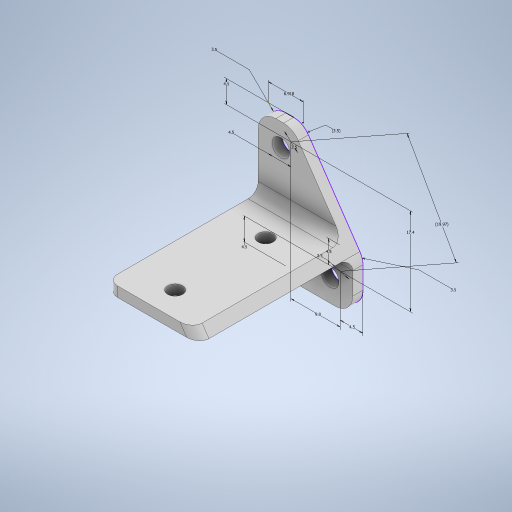
# Autodesk Inventor part: BLTouch Mount
Saved by Autodesk Inventor 2023 (Build 270158000, 158)
## iProperties
Created: 2024-01-21
Part Number: BLTouch Mount
Material: Generic
Document SubType Name: Modeling
Designer: Lyall
Density: 1 g/cm^3
Appearance: Default
Author: Lyall
Autodesk Inventor part; units mm, degrees
note: some values were not read from the file. Chosen so that the rebuilt part matches the saved one: edges of "Fillet2".
ref_plane "YZ Plane" through (0, 0, 0) normal (1, 0, 0) x (0, 1, 0)
ref_plane "XZ Plane" through (0, 0, 0) normal (0, 1, 0) x (-1, 0, 0)
ref_plane "XY Plane" through (0, 0, 0) normal (0, 0, 1) x (1, 0, 0)
sketch "Sketch1" plane through (0, 0, 0) normal (0, 0, 1) x (1, 0, 0)
  circle A0 centre (4.5, -4.5) radius 1.75
  circle A1 centre (14.3, -21.9) radius 1.75
  line L0 (15.3, -26.4) -> (3.5, -26.4)
  line L1 (0, -22.9) -> (0, -3.5)
  line L2 (18.8, -22.9) -> (18.8, -19.7088)
  line L3 (5.0373, 0) -> (3.5, 0)
  arc A2 (3.5, 0) -> (0, -3.5) centre (3.5, -3.5) ccw
  arc A3 (7.956, -1.5683) -> (5.0373, 0) centre (5.0373, -3.5) ccw
  arc A4 (15.3, -26.4) -> (18.8, -22.9) centre (15.3, -22.9) ccw
  arc A5 (0, -22.9) -> (3.5, -26.4) centre (3.5, -22.9) ccw
  line L4 (14.3, -21.9) -> (14.3, -17.4)
  line L5 (18.8, -19.7088) -> (18.8, -18.5234)
  line L6 (18.19, -16.5491) -> (7.956, -1.5683)
  arc A6 (18.8, -18.5234) -> (18.19, -16.5491) centre (15.3, -18.5234) ccw
  point P0 (0, 0)
  point P1 (6.9181, 0)
  point P2 (4.2687, 0)
  dimension "d0" = 3.5
  dimension "d1" = 3.5
  dimension "d34" = 4.5
  dimension "d35" = 4.5
  dimension "d38" = 6.9181
  dimension "d39" = 3.5
  dimension "d46" = 3.5
  dimension "d66" = 9.8
  dimension "d67" = 17.4
  dimension "d68" = 19.97
  dimension "d69" = 4.5
  dimension "d70" = 4.5
  dimension "d71" = 4.5
  dimension "d72" = 3.5
  constraints: 14 end point, 10 point on circle, 9 tangent, 7 centre point, 3 equal radius, 3 point on line, 3 vertical, 1 horizontal, 1 midpoint
  measures "d0" diameter of A0
  measures "d1" diameter of A1
  measures "d34" distance from line of L1 A0.centre
  measures "d35" distance from line of L0 L4.start
  measures "d38" distance of point (6.918, 0) point (0, 0)
  measures "d39" radius of A2
  measures "d46" radius of A3
  measures "d66" horizontal distance of L4.start A0.centre
  measures "d67" vertical distance of A0.centre L4.start
  measures "d68" distance of L4.start A0.centre
  measures "d69" distance from line of L4.start L2
  measures "d70" vertical distance of point (4.269, 0) A0.centre
  measures "d71" distance of L4.start L4.end
  measures "d72" radius of A6
extrude "Extrusion5" add sketch "Sketch1" along normal blind 2
sketch "Sketch5" plane through (0, 0, 2) normal (0, 0, 1) x (1, 0, 0)
  line L0 (0, -3.5) -> (0, -22.9) projected
  line L1 (0, -14.5491) -> (16.1836, -14.5491)
  line L2 (0, -14.5491) -> (0, -16.5491)
  line L3 (0, -16.5491) -> (17.3511, -16.5491)
  line L4 (0, -14.5491) -> (16.8237, -14.5491)
  line L5 (18.19, -16.5491) -> (7.956, -1.5683) projected
  line L6 (18.19, -16.5491) -> (0, -16.5491)
  line L7 (0, -3.5) -> (0, -22.9) projected
  line L8 (18.19, -16.5491) -> (16.8237, -14.5491)
  point P0 (0, 0)
  point P1 (0, -16.5491)
  dimension "d42" = 2
  dimension "d76" = 0
  constraints: 12 end point, 3 horizontal, 3 point on line, 2 perpendicular, 1 collinear
  measures "d42" distance of L1.start L2.end
  measures "d76" distance from line of L5.start L6
extrude "Extrusion6" add sketch "Sketch5" along normal blind 30
fillet "Fillet2" radius 2 3 edges at (0, -15.5491, 32) (8.4119, -14.5491, 2) (9.095, -16.5491, 2)
sketch "Sketch6" plane through (0, -22.9, 0) normal (-1, 0, 0) x (0, 0, 1)
  line L0 (4, 6.3509) -> (30, 6.3509) projected
  line L1 (2, 2.75) -> (2, -0.75) projected
  line L2 (2, 6.3509) -> (2, 1.3509)
  line L3 (2, 6.3509) -> (2, 1.3509)
  line L4 (2, 1.3509) -> (21.3649, 6.3509)
  line L5 (21.3649, 6.3509) -> (2, 6.3509)
  point P0 (0, 22.9)
  point P1 (2, 2.75)
  dimension "d73" = 5
  dimension "d74" = 5
  dimension "d75" = 20
  constraints: 8 end point, 2 point on line, 1 collinear, 1 perpendicular
  measures "d73" distance of L2.start L2.end
  measures "d74" distance of L2.start L2.end
  measures "d75" distance of L2.end L4.end
extrude "Extrusion7" add sketch "Sketch6" against normal blind 2
sketch "Sketch7" plane through (0, -14.5491, 4) normal (0, 1, 0) x (1, 0, 0)
  circle A0 centre (8.4575, -5) radius 1.5
  circle A1 centre (8.4575, -23) radius 1.5
  line L0 (0, 0) -> (0, -26) projected
  line L1 (16.8237, -28) -> (2, -28) projected
  line L2 (0, 0) -> (16.8237, 0) projected
  line L3 (16.8237, 0) -> (16.8237, -28) projected
  point P0 (0, 4)
  point P1 (13.7853, -28)
  dimension "d54" = 3
  dimension "d55" = 3
  dimension "d56" = 18
  dimension "d58" = 8.4575
  dimension "d59" = 8.4575
  dimension "d62" = 5
  dimension "d63" = 5
  dimension "d78" = 16.8237
  constraints: 2 centre point
  measures "d54" diameter of A0
  measures "d55" diameter of A1
  measures "d56" distance of A0.centre A1.centre
  measures "d58" distance from line of L0 A1.centre
  measures "d59" distance from line of L0 A0.centre
  measures "d62" distance from line of L1 A1.centre
  measures "d63" distance from line of L2 A0.centre
  measures "d78" distance between parallel lines of L0 L3
extrude "Extrusion8" cut sketch "Sketch7" against normal blind 2
fillet "Fillet3" radius 2 1 edges at (17.5069, -15.5491, 32)
body "Solid1"
